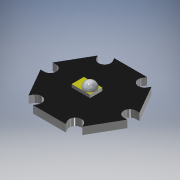
# Autodesk Inventor part: Luxeon Rebel Star
Saved by Autodesk Inventor 2017 (Build 210142000, 142)
## iProperties
Created: 2014-06-11
Part Number: Luxeon Rebel Star
Material: Allgemein
Document SubType Name: Modeling
Designer: Merges
Density: 1 g/cm^3
Appearance: Vorgabe
Author: Merges
Autodesk Inventor part; units mm, degrees
ref_plane "YZ Plane" through (0, 0, 0) normal (1, 0, 0) x (0, 1, 0)
ref_plane "XZ Plane" through (0, 0, 0) normal (0, 1, 0) x (-1, 0, 0)
ref_plane "XY Plane" through (0, 0, 0) normal (0, 0, 1) x (1, 0, 0)
sketch "Skizze1" plane through (0, 0, 0) normal (0, 0, 1) x (1, 0, 0)
  line L0 (-3, 1.5) -> (1.5, 1.5)
  line L1 (1.5, 1.5) -> (1.5, -1.5)
  line L2 (-3, -1.5) -> (-3, 1.5)
  line L3 (1.5, 1.5) -> (-1.5, -1.5) construction
  line L4 (-1.5, -1.5) -> (1.5, -1.5) construction
  line L5 (0, 0) -> (0.1963, -0.4081) construction
  line L6 (-3, -1.5) -> (1.5, -1.5)
  dimension "d0" = 3
  dimension "d1" = 4.5
  constraints: 14 end point, 3 perpendicular, 1 collinear, 1 horizontal, 1 midpoint, 1 parallel, 1 other
  measures "d0" distance of L0.end L1.end
  measures "d1" distance of L1.end L2.start
extrude "Extrusion1" add sketch "Skizze1" against normal blind 0.75
sketch "Skizze2" plane through (0, 0, 0) normal (1, 0, 0) x (0, 1, 0)
  line L0 (-1.5, 0) -> (1.5, 0) projected
  arc A0 (0, 1.5) -> (-1.5, 0) centre (0, 0) ccw
  line L1 (0, 0) -> (0, 1.5)
  line L2 (0, 0) -> (-1.5, 0)
  dimension "d4" = 1.5
  constraints: 4 end point, 2 point on circle, 1 centre point, 1 coincident, 1 collinear, 1 perpendicular, 1 point on line
  measures "d4" radius of A0
revolve "Umdrehung1" add sketch "Skizze2" angle 360 about axis through (0, 0, 0) along (0, 0, 1)
sketch "Skizze3" plane through (0, 0, -0.75) normal (0, 0, -1) x (-1, 0, 0)
  line L0 (11.4893, 0) -> (5.7446, -9.95)
  line L1 (5.7446, -9.95) -> (-5.7446, -9.95)
  line L2 (-5.7446, -9.95) -> (-11.4893, 0)
  line L3 (-11.4893, 0) -> (-5.7446, 9.95)
  line L4 (-5.7446, 9.95) -> (5.7446, 9.95)
  line L5 (5.7446, 9.95) -> (11.4893, 0)
  point P0 (0, 0)
  point P1 (0, 0)
  dimension "d7" = 19.9
  constraints: 12 end point, 1 coincident, 1 horizontal, 13 other
  measures "d7" distance between parallel lines of L4 L1
extrude "Extrusion2" add sketch "Skizze3" along normal blind 1.8
sketch "Skizze4" plane through (0, 0, -0.75) normal (0, 0, 1) x (1, 0, 0)
  line L0 (-11.4893, 0) -> (-5.7446, -9.95) projected
  line L1 (-5.7446, 9.95) -> (-11.4893, 0) projected
  line L2 (1.5, -1.5) -> (-3, -1.5) projected
  line L3 (0, 0) -> (-9.77, 0) construction
  arc A0 (-9.77, -1.5) -> (-9.77, 1.5) centre (-9.77, 0) ccw
  line L4 (-9.77, -1.5) -> (-10.6232, -1.5)
  line L5 (-9.77, 1.5) -> (-10.6232, 1.5)
  dimension "d10" = 9.77
  dimension "d11" = 3
  constraints: 6 end point, 3 parallel, 2 point on circle, 2 point on line, 1 centre point, 1 coincident, 1 tangent
  measures "d10" distance of L3.start L3.end
  measures "d11" distance between parallel lines of L5 L4
extrude "Extrusion3" cut sketch "Skizze4" against normal blind 1.8
pattern_circular "Runde Anordnung1" count 6 over 360 about axis through (0, 0, -10) along (0, 0, 1) of "Extrusion3"
